Autodesk Fusion 360 part; units mm, degrees
note: some values were not read from the file. Set by a fixed rule: which sketch regions a step uses.
(part 6 of 15)
  line L4345 (-60.2725, -88.9984) -> (-60.4916, -88.82)
  line L4346 (182.212, -88.6982) -> (182.013, -88.8773)
  line L4347 (180.093, -85.6323) -> (180.347, -85.5433)
  line L4348 (-53.9287, -87.3136) -> (-53.7516, -87.3685)
  line L4349 (182.709, -87.7613) -> (182.636, -88.0196)
  line L4350 (182.744, -87.4953) -> (182.709, -87.7613)
  line L4351 (181.547, -89.1426) -> (181.292, -89.2235)
  line L4352 (181.891, -85.788) -> (182.104, -85.9508)
  line L4353 (181.789, -89.0264) -> (181.547, -89.1426)
  line L4354 (-58.9343, -89.3532) -> (-59.2167, -89.3599)
  line L4355 (181.657, -85.6568) -> (181.891, -85.788)
  line L4356 (182.636, -88.0196) -> (182.527, -88.2651)
  line L4357 (182.58, -86.5941) -> (182.673, -86.8459)
  line L4358 (-60.6018, -86.0161) -> (-60.3974, -85.8211)
  line L4359 (182.452, -86.3579) -> (182.58, -86.5941)
  line L4360 (182.293, -86.142) -> (182.452, -86.3579)
  line L4361 (-57.8967, -88.9424) -> (-58.1316, -89.0994)
  line L4362 (-58.1316, -89.0994) -> (-58.3863, -89.2216)
  line L4363 (182.527, -88.2651) -> (182.385, -88.4928)
  line L4364 (178.949, -87.3163) -> (178.976, -87.0493)
  line L4365 (-59.9168, -85.5266) -> (-59.6503, -85.433)
  line L4366 (-53.7516, -87.3685) -> (-53.5885, -87.4566)
  line L4367 (181.292, -89.2235) -> (181.027, -89.2676)
  line L4368 (-53.5885, -87.4566) -> (-53.4456, -87.5748)
  line L4369 (179.277, -86.308) -> (179.443, -86.0973)
  line L4370 (-61.0246, -86.7441) -> (-60.9186, -86.4822)
  line L4371 (182.673, -86.8459) -> (182.729, -87.1083)
  line L4372 (-58.3863, -89.2216) -> (-58.6556, -89.3068)
  line L4373 (-60.4916, -88.82) -> (-60.6834, -88.6126)
  line L4374 (182.385, -88.4928) -> (182.212, -88.6982)
  line L4375 (-59.2167, -89.3599) -> (-59.4973, -89.3267)
  line L4376 (182.013, -88.8773) -> (181.789, -89.0264)
  line L4377 (252.733, -84.9451) -> (252.831, -85.2102)
  line L4378 (252.792, -86.4456) -> (252.678, -86.704)
  line L4379 (-54.3237, -89.1721) -> (-54.5, -89.1148)
  line L4380 (-54.2977, -87.311) -> (-54.1131, -87.2942)
  line L4381 (251.901, -87.5054) -> (251.647, -87.6277)
  line L4382 (252.528, -86.9437) -> (252.347, -87.16)
  line L4383 (-53.6107, -89.0463) -> (-53.7762, -89.1299)
  line L4384 (-54.9182, -88.7588) -> (-55.003, -88.5939)
  line L4385 (249.541, -87.2261) -> (249.349, -87.0187)
  line L4386 (-54.7844, -87.5655) -> (-54.6399, -87.4493)
  line L4387 (249.349, -87.0187) -> (249.189, -86.7863)
  line L4388 (249.008, -85.1501) -> (249.114, -84.8883)
  line L4389 (252.136, -87.3485) -> (251.901, -87.5054)
  line L4390 (252.008, -84.0966) -> (252.233, -84.268)
  line L4391 (-54.5, -89.1148) -> (-54.6619, -89.0243)
  line L4392 (249.431, -84.4221) -> (249.635, -84.2271)
  line L4393 (249.865, -84.0629) -> (250.116, -83.9327)
  line L4394 (-55.0696, -88.231) -> (-55.0489, -88.0467)
  line L4395 (252.678, -86.704) -> (252.528, -86.9437)
  line L4396 (-53.3284, -87.7185) -> (-53.2414, -87.8822)
  line L4397 (252.831, -85.2102) -> (252.89, -85.4864)
  line L4398 (-54.4756, -87.3634) -> (-54.2977, -87.311)
  line L4399 (252.89, -85.4864) -> (252.91, -85.7682)
  line L4400 (-54.9929, -87.87) -> (-54.9036, -87.7075)
  line L4401 (251.498, -83.8566) -> (251.762, -83.9585)
  line L4402 (-54.6399, -87.4493) -> (-54.4756, -87.3634)
  line L4403 (251.377, -87.7129) -> (251.099, -87.7593)
  line L4404 (249.114, -84.8883) -> (249.256, -84.644)
  line L4405 (249.256, -84.644) -> (249.431, -84.4221)
  line L4406 (-53.2414, -87.8822) -> (-53.1878, -88.0597)
  line L4407 (248.922, -85.9876) -> (248.911, -85.7054)
  line L4408 (178.976, -87.0493) -> (179.041, -86.7889)
  line L4409 (252.869, -86.1737) -> (252.792, -86.4456)
  line L4410 (-53.1933, -88.4547) -> (-53.2518, -88.6306)
  line L4411 (-54.8031, -88.9041) -> (-54.9182, -88.7588)
  line L4412 (251.223, -83.7928) -> (251.498, -83.8566)
  line L4413 (251.647, -87.6277) -> (251.377, -87.7129)
  line L4414 (-53.1878, -88.0597) -> (-53.1697, -88.2442)
  line L4415 (-53.4456, -87.5748) -> (-53.3284, -87.7185)
  line L4416 (-55.0489, -88.0467) -> (-54.9929, -87.87)
  line L4417 (-55.0541, -88.4157) -> (-55.0696, -88.231)
  line L4418 (252.91, -85.7682) -> (252.906, -85.8938)
  line L4419 (252.906, -85.8938) -> (252.869, -86.1737)
  line L4420 (-54.6619, -89.0243) -> (-54.8031, -88.9041)
  line L4421 (251.762, -83.9585) -> (252.008, -84.0966)
  line L4422 (248.911, -85.7054) -> (248.94, -85.4243)
  line L4423 (-55.003, -88.5939) -> (-55.0541, -88.4157)
  line L4424 (-53.9547, -89.1798) -> (-54.1396, -89.194)
  line L4425 (252.431, -84.4693) -> (252.599, -84.6965)
  line L4426 (-54.9036, -87.7075) -> (-54.7844, -87.5655)
  line L4427 (248.94, -85.4243) -> (249.008, -85.1501)
  line L4428 (179.213, -88.3432) -> (179.093, -88.1031)
  line L4429 (-53.4646, -88.9322) -> (-53.6107, -89.0463)
  line L4430 (-53.7762, -89.1299) -> (-53.9547, -89.1798)
  line L4431 (-53.2518, -88.6306) -> (-53.3434, -88.7918)
  line L4432 (-53.1697, -88.2442) -> (-53.1701, -88.2707)
  line L4433 (180.347, -85.5433) -> (180.61, -85.491)
  line L4434 (252.233, -84.268) -> (252.431, -84.4693)
  line L4435 (252.599, -84.6965) -> (252.733, -84.9451)
  line L4436 (179.637, -85.912) -> (179.855, -85.756)
  line L4437 (-54.1131, -87.2942) -> (-53.9287, -87.3136)
  line L4438 (-53.1701, -88.2707) -> (-53.1933, -88.4547)
  line L4439 (-54.1396, -89.194) -> (-54.3237, -89.1721)
  line L4440 (85.4442, -85.7281) -> (85.4402, -85.8537)
  line L4441 (84.2957, -83.9185) -> (84.5422, -84.0565)
  line L4442 (82.5362, -87.5101) -> (82.2941, -87.3644)
  line L4443 (81.507, -86.2255) -> (81.4562, -85.9476)
  line L4444 (252.347, -87.16) -> (252.136, -87.3485)
  line L4445 (250.66, -83.7839) -> (250.942, -83.7684)
  line L4446 (84.8804, -87.1199) -> (84.67, -87.3084)
  line L4447 (249.063, -86.5335) -> (248.973, -86.2656)
  line L4448 (82.1693, -84.1871) -> (82.3992, -84.0228)
  line L4449 (251.099, -87.7593) -> (250.816, -87.766)
  line L4450 (81.5964, -86.4935) -> (81.507, -86.2255)
  line L4451 (246.072, -87.5859) -> (245.888, -87.6001)
  line L4452 (250.002, -87.5502) -> (249.76, -87.4045)
  line L4453 (246.684, -87.1979) -> (246.563, -87.3383)
  line L4454 (246.251, -87.536) -> (246.072, -87.5859)
  line L4455 (245.704, -87.5781) -> (245.527, -87.5209)
  line L4456 (245.365, -87.4304) -> (245.224, -87.3102)
  line L4457 (84.7668, -84.2279) -> (84.965, -84.4292)
  line L4458 (82.2941, -87.3644) -> (82.0751, -87.186)
  line L4459 (84.1804, -87.5877) -> (83.9111, -87.6728)
  line L4460 (85.267, -84.9051) -> (85.3647, -85.1701)
  line L4461 (85.4402, -85.8537) -> (85.4026, -86.1337)
  line L4462 (82.7963, -87.6203) -> (82.5362, -87.5101)
  line L4463 (84.4351, -87.4654) -> (84.1804, -87.5877)
  line L4464 (85.3647, -85.1701) -> (85.4242, -85.4463)
  line L4465 (249.189, -86.7863) -> (249.063, -86.5335)
  line L4466 (85.4026, -86.1337) -> (85.3259, -86.4056)
  line L4467 (85.0622, -86.9037) -> (84.8804, -87.1199)
  line L4468 (83.757, -83.7527) -> (84.0322, -83.8165)
  line L4469 (250.116, -83.9327) -> (250.383, -83.8391)
  line L4470 (84.5422, -84.0565) -> (84.7668, -84.2279)
  line L4471 (81.7227, -86.7462) -> (81.5964, -86.4935)
  line L4472 (84.965, -84.4292) -> (85.1328, -84.6565)
  line L4473 (246.834, -86.8608) -> (246.775, -87.0367)
  line L4474 (246.439, -85.8627) -> (246.582, -85.9809)
  line L4475 (83.9111, -87.6728) -> (83.6324, -87.7192)
  line L4476 (85.1328, -84.6565) -> (85.267, -84.9051)
  line L4477 (250.536, -87.7327) -> (250.263, -87.6603)
  line L4478 (250.263, -87.6603) -> (250.002, -87.5502)
  line L4479 (84.67, -87.3084) -> (84.4351, -87.4654)
  line L4480 (81.4451, -85.6653) -> (81.4739, -85.3842)
  line L4481 (85.2117, -86.664) -> (85.0622, -86.9037)
  line L4482 (81.6481, -84.8482) -> (81.79, -84.6039)
  line L4483 (246.699, -86.1246) -> (246.786, -86.2883)
  line L4484 (84.0322, -83.8165) -> (84.2957, -83.9185)
  line L4485 (250.942, -83.7684) -> (251.223, -83.7928)
  line L4486 (249.76, -87.4045) -> (249.541, -87.2261)
  line L4487 (85.4242, -85.4463) -> (85.4442, -85.7281)
  line L4488 (250.816, -87.766) -> (250.536, -87.7327)
  line L4489 (83.0694, -87.6927) -> (82.7963, -87.6203)
  line L4490 (83.3499, -87.7259) -> (83.0694, -87.6927)
  line L4491 (85.3259, -86.4056) -> (85.2117, -86.664)
  line L4492 (81.4562, -85.9476) -> (81.4451, -85.6653)
  line L4493 (83.6324, -87.7192) -> (83.3499, -87.7259)
  line L4494 (82.0751, -87.186) -> (81.8833, -86.9786)
  line L4495 (246.582, -85.9809) -> (246.699, -86.1246)
  line L4496 (81.9649, -84.3821) -> (82.1693, -84.1871)
  line L4497 (248.973, -86.2656) -> (248.922, -85.9876)
  line L4498 (81.8833, -86.9786) -> (81.7227, -86.7462)
  line L4499 (246.839, -86.4658) -> (246.858, -86.6503)
  line L4500 (249.635, -84.2271) -> (249.865, -84.0629)
  line L4501 (250.383, -83.8391) -> (250.66, -83.7839)
  line L4502 (89.3966, -86.6368) -> (89.3734, -86.8207)
  line L4503 (89.1211, -85.9408) -> (89.2383, -86.0845)
  line L4504 (245.527, -87.5209) -> (245.365, -87.4304)
  line L4505 (245.73, -85.7171) -> (245.914, -85.7003)
  line L4506 (81.542, -85.1101) -> (81.6481, -84.8482)
  line L4507 (244.973, -86.8218) -> (244.958, -86.637)
  line L4508 (89.1021, -87.2982) -> (88.956, -87.4124)
  line L4509 (245.109, -87.1649) -> (245.024, -87)
  line L4510 (245.224, -87.3102) -> (245.109, -87.1649)
  line L4511 (88.6119, -87.5458) -> (88.4271, -87.56)
  line L4512 (245.124, -86.1136) -> (245.243, -85.9716)
  line L4513 (83.1935, -83.7439) -> (83.4756, -83.7284)
  line L4514 (88.243, -87.5381) -> (88.0666, -87.4808)
  line L4515 (89.397, -86.6102) -> (89.3966, -86.6368)
  line L4516 (245.914, -85.7003) -> (246.099, -85.7197)
  line L4517 (244.958, -86.637) -> (244.978, -86.4528)
  line L4518 (88.8151, -85.7345) -> (88.9782, -85.8227)
  line L4519 (245.552, -85.7695) -> (245.73, -85.7171)
  line L4520 (89.2383, -86.0845) -> (89.3253, -86.2482)
  line L4521 (89.3789, -86.4257) -> (89.397, -86.6102)
  line L4522 (89.3148, -86.9966) -> (89.2233, -87.1579)
  line L4523 (82.6499, -83.8926) -> (82.9164, -83.799)
  line L4524 (87.9048, -87.3903) -> (87.7636, -87.2702)
  line L4525 (88.0666, -87.4808) -> (87.9048, -87.3903)
  line L4526 (-63.7818, -87.3657) -> (-63.9604, -87.4155)
  line L4527 (89.2233, -87.1579) -> (89.1021, -87.2982)
  line L4528 (88.956, -87.4124) -> (88.7905, -87.4959)
  line L4529 (88.7905, -87.4959) -> (88.6119, -87.5458)
  line L4530 (81.79, -84.6039) -> (81.9649, -84.3821)
  line L4531 (244.978, -86.4528) -> (245.034, -86.2761)
  line L4532 (-63.7572, -85.6042) -> (-63.5941, -85.6924)
  line L4533 (82.9164, -83.799) -> (83.1935, -83.7439)
  line L4534 (246.417, -87.4524) -> (246.251, -87.536)
  line L4535 (81.4739, -85.3842) -> (81.542, -85.1101)
  line L4536 (87.7636, -87.2702) -> (87.6484, -87.1249)
  line L4537 (-63.9604, -87.4155) -> (-64.1452, -87.4297)
  line L4538 (-64.1452, -87.4297) -> (-64.3293, -87.4078)
  line L4539 (245.387, -85.8554) -> (245.552, -85.7695)
  line L4540 (245.024, -87) -> (244.973, -86.8218)
  line L4541 (88.4271, -87.56) -> (88.243, -87.5381)
  line L4542 (-63.1757, -86.5065) -> (-63.199, -86.6904)
  line L4543 (87.6631, -86.0735) -> (87.7823, -85.9315)
  line L4544 (-63.199, -86.6904) -> (-63.2575, -86.8664)
  line L4545 (-63.6163, -87.2821) -> (-63.7818, -87.3657)
  line L4546 (88.638, -85.6796) -> (88.8151, -85.7345)
  line L4547 (246.857, -86.6768) -> (246.834, -86.8608)
  line L4548 (246.563, -87.3383) -> (246.417, -87.4524)
  line L4549 (246.099, -85.7197) -> (246.276, -85.7745)
  line L4550 (245.243, -85.9716) -> (245.387, -85.8554)
  line L4551 (88.9782, -85.8227) -> (89.1211, -85.9408)
  line L4552 (-64.3293, -87.4078) -> (-64.5057, -87.3505)
  line L4553 (-64.5057, -87.3505) -> (-64.6675, -87.26)
  line L4554 (245.888, -87.6001) -> (245.704, -87.5781)
  line L4555 (89.3734, -86.8207) -> (89.3148, -86.9966)
  line L4556 (-63.9343, -85.5494) -> (-63.7572, -85.6042)
  line L4557 (87.5126, -86.7817) -> (87.4971, -86.597)
  line L4558 (246.775, -87.0367) -> (246.684, -87.1979)
  line L4559 (82.3992, -84.0228) -> (82.6499, -83.8926)
  line L4560 (245.034, -86.2761) -> (245.124, -86.1136)
  line L4561 (246.858, -86.6503) -> (246.857, -86.6768)
  line L4562 (246.276, -85.7745) -> (246.439, -85.8627)
  line L4563 (83.4756, -83.7284) -> (83.757, -83.7527)
  line L4564 (89.3253, -86.2482) -> (89.3789, -86.4257)
  line L4565 (246.786, -86.2883) -> (246.839, -86.4658)
  line L4566 (270.656, -82.7999) -> (270.919, -82.9018)
  line L4567 (-64.1187, -85.53) -> (-63.9343, -85.5494)
  line L4568 (271.391, -83.2112) -> (271.589, -83.4125)
  line L4569 (268.131, -85.2088) -> (268.08, -84.9309)
  line L4570 (272.064, -84.837) -> (272.026, -85.117)
  line L4571 (271.686, -85.887) -> (271.504, -86.1033)
  line L4572 (-63.3341, -85.9542) -> (-63.247, -86.1179)
  line L4573 (65.1382, -82.8617) -> (65.3847, -82.9998)
  line L4574 (-64.9985, -86.1057) -> (-64.9092, -85.9432)
  line L4575 (-65.0086, -86.8297) -> (-65.0597, -86.6514)
  line L4576 (268.08, -84.9309) -> (268.069, -84.6486)
  line L4577 (-64.3034, -85.5468) -> (-64.1187, -85.53)
  line L4578 (270.099, -82.7117) -> (270.381, -82.7361)
  line L4579 (65.3847, -82.9998) -> (65.6092, -83.1712)
  line L4580 (87.9268, -85.8153) -> (88.0911, -85.7294)
  line L4581 (272.026, -85.117) -> (271.95, -85.3889)
  line L4582 (-65.0753, -86.4667) -> (-65.0546, -86.2824)
  line L4583 (-63.2575, -86.8664) -> (-63.3491, -87.0276)
  line L4584 (87.7823, -85.9315) -> (87.9268, -85.8153)
  line L4585 (88.4536, -85.6603) -> (88.638, -85.6796)
  line L4586 (271.891, -83.8884) -> (271.988, -84.1535)
  line L4587 (-64.9092, -85.9432) -> (-64.79, -85.8012)
  line L4588 (64.5995, -82.696) -> (64.8747, -82.7598)
  line L4589 (269.693, -86.676) -> (269.42, -86.6036)
  line L4590 (-63.5941, -85.6924) -> (-63.4513, -85.8106)
  line L4591 (268.918, -86.3477) -> (268.699, -86.1694)
  line L4592 (271.504, -86.1033) -> (271.294, -86.2918)
  line L4593 (270.256, -86.7026) -> (269.974, -86.7092)
  line L4594 (-64.79, -85.8012) -> (-64.6455, -85.685)
  line L4595 (-64.6675, -87.26) -> (-64.8087, -87.1399)
  line L4596 (-63.4513, -85.8106) -> (-63.3341, -85.9542)
  line L4597 (87.4971, -86.597) -> (87.5177, -86.4127)
  line L4598 (87.5738, -86.236) -> (87.6631, -86.0735)
  line L4599 (87.6484, -87.1249) -> (87.5637, -86.96)
  line L4600 (-64.8087, -87.1399) -> (-64.9239, -86.9946)
  line L4601 (-64.9239, -86.9946) -> (-65.0086, -86.8297)
  line L4602 (87.5177, -86.4127) -> (87.5738, -86.236)
  line L4603 (-65.0546, -86.2824) -> (-64.9985, -86.1057)
  line L4604 (272.048, -84.4296) -> (272.068, -84.7114)
  line L4605 (271.294, -86.2918) -> (271.059, -86.4487)
  line L4606 (269.42, -86.6036) -> (269.16, -86.4935)
  line L4607 (271.95, -85.3889) -> (271.835, -85.6473)
  line L4608 (-63.1753, -86.48) -> (-63.1757, -86.5065)
  line L4609 (88.269, -85.6771) -> (88.4536, -85.6603)
  line L4610 (88.0911, -85.7294) -> (88.269, -85.6771)
  line L4611 (-63.4702, -87.1679) -> (-63.6163, -87.2821)
  line L4612 (271.757, -83.6398) -> (271.891, -83.8884)
  line L4613 (270.381, -82.7361) -> (270.656, -82.7999)
  line L4614 (-63.247, -86.1179) -> (-63.1934, -86.2954)
  line L4615 (270.919, -82.9018) -> (271.166, -83.0398)
  line L4616 (272.068, -84.7114) -> (272.064, -84.837)
  line L4617 (271.835, -85.6473) -> (271.686, -85.887)
  line L4618 (-65.0597, -86.6514) -> (-65.0753, -86.4667)
  line L4619 (271.988, -84.1535) -> (272.048, -84.4296)
  line L4620 (-63.1934, -86.2954) -> (-63.1753, -86.48)
  line L4621 (268.272, -83.8316) -> (268.414, -83.5873)
  line L4622 (64.8747, -82.7598) -> (65.1382, -82.8617)
  line L4623 (271.166, -83.0398) -> (271.391, -83.2112)
  line L4624 (269.274, -82.8759) -> (269.54, -82.7823)
  line L4625 (271.589, -83.4125) -> (271.757, -83.6398)
  line L4626 (-63.3491, -87.0276) -> (-63.4702, -87.1679)
  line L4627 (87.5637, -86.96) -> (87.5126, -86.7817)
  line L4628 (-64.4812, -85.5991) -> (-64.3034, -85.5468)
  line L4629 (-64.6455, -85.685) -> (-64.4812, -85.5991)
  line L4630 (66.2072, -84.1134) -> (66.2667, -84.3896)
  line L4631 (269.817, -82.7272) -> (270.099, -82.7117)
  line L4632 (63.1366, -86.3077) -> (62.9175, -86.1293)
  line L4633 (62.4389, -85.4367) -> (62.3494, -85.1688)
  line L4634 (62.5651, -85.6895) -> (62.4389, -85.4367)
  line L4635 (268.346, -85.7295) -> (268.22, -85.4768)
  line L4636 (270.804, -86.571) -> (270.535, -86.6562)
  line L4637 (65.6092, -83.1712) -> (65.8074, -83.3725)
  line L4638 (270.535, -86.6562) -> (270.256, -86.7026)
  line L4639 (65.9753, -83.5997) -> (66.1094, -83.8484)
  line L4640 (62.4906, -83.7915) -> (62.6324, -83.5472)
  line L4641 (65.8074, -83.3725) -> (65.9753, -83.5997)
  line L4642 (66.1094, -83.8484) -> (66.2072, -84.1134)
  line L4643 (268.22, -85.4768) -> (268.131, -85.2088)
  line L4644 (62.3164, -84.3275) -> (62.3845, -84.0533)
  line L4645 (66.2451, -85.077) -> (66.1684, -85.3489)
  line L4646 (66.0541, -85.6072) -> (65.9046, -85.847)
  line L4647 (64.1924, -86.6692) -> (63.9118, -86.636)
  line L4648 (62.3845, -84.0533) -> (62.4906, -83.7915)
  line L4649 (62.3494, -85.1688) -> (62.2987, -84.8908)
  line L4650 (64.7535, -86.6161) -> (64.4748, -86.6625)
  line L4651 (271.059, -86.4487) -> (270.804, -86.571)
  line L4652 (62.6324, -83.5472) -> (62.8073, -83.3254)
  line L4653 (265.256, -84.663) -> (265.433, -84.7178)
  line L4654 (65.9046, -85.847) -> (65.7229, -86.0632)
  line L4655 (64.4748, -86.6625) -> (64.1924, -86.6692)
  line L4656 (268.069, -84.6486) -> (268.098, -84.3676)
  line L4657 (268.793, -83.1704) -> (269.023, -83.0062)
  line L4658 (62.8073, -83.3254) -> (63.0118, -83.1304)
  line L4659 (63.4923, -82.8359) -> (63.7589, -82.7423)
  line L4660 (62.2987, -84.8908) -> (62.2876, -84.6086)
  line L4661 (65.7229, -86.0632) -> (65.5124, -86.2517)
  line L4662 (66.2866, -84.6714) -> (66.2827, -84.797)
  line L4663 (63.3786, -86.4534) -> (63.1366, -86.3077)
  line L4664 (265.841, -86.1412) -> (265.72, -86.2815)
  line L4665 (265.72, -86.2815) -> (265.574, -86.3957)
  line L4666 (62.7257, -85.9219) -> (62.5651, -85.6895)
  line L4667 (268.414, -83.5873) -> (268.589, -83.3654)
  line L4668 (269.974, -86.7092) -> (269.693, -86.676)
  line L4669 (65.0229, -86.5309) -> (64.7535, -86.6161)
  line L4670 (65.2775, -86.4086) -> (65.0229, -86.5309)
  line L4671 (66.2667, -84.3896) -> (66.2866, -84.6714)
  line L4672 (66.1684, -85.3489) -> (66.0541, -85.6072)
  line L4673 (63.9118, -86.636) -> (63.6388, -86.5636)
  line L4674 (66.2827, -84.797) -> (66.2451, -85.077)
  line L4675 (268.098, -84.3676) -> (268.166, -84.0934)
  line L4676 (268.507, -85.9619) -> (268.346, -85.7295)
  line L4677 (62.2876, -84.6086) -> (62.3164, -84.3275)
  line L4678 (62.9175, -86.1293) -> (62.7257, -85.9219)
  line L4679 (265.409, -86.4793) -> (265.23, -86.5291)
  line L4680 (64.318, -82.6716) -> (64.5995, -82.696)
  line L4681 (265.997, -85.4091) -> (266.015, -85.5936)
  line L4682 (64.0359, -82.6872) -> (64.318, -82.6716)
  line L4683 (269.16, -86.4935) -> (268.918, -86.3477)
  line L4684 (63.2416, -82.9661) -> (63.4923, -82.8359)
  line L4685 (264.685, -86.4641) -> (264.523, -86.3737)
  line L4686 (269.54, -82.7823) -> (269.817, -82.7272)
  line L4687 (264.523, -86.3737) -> (264.382, -86.2535)
  line L4688 (65.5124, -86.2517) -> (65.2775, -86.4086)
  line L4689 (63.6388, -86.5636) -> (63.3786, -86.4534)
  line L4690 (268.699, -86.1694) -> (268.507, -85.9619)
  line L4691 (268.166, -84.0934) -> (268.272, -83.8316)
  line L4692 (268.589, -83.3654) -> (268.793, -83.1704)
  line L4693 (269.023, -83.0062) -> (269.274, -82.8759)
  line L4694 (265.856, -85.0679) -> (265.943, -85.2316)
  line L4695 (265.991, -85.804) -> (265.933, -85.98)
  line L4696 (265.23, -86.5291) -> (265.045, -86.5434)
  line L4697 (265.933, -85.98) -> (265.841, -86.1412)
  line L4698 (63.0118, -83.1304) -> (63.2416, -82.9661)
  line L4699 (265.943, -85.2316) -> (265.997, -85.4091)
  line L4700 (266.015, -85.5936) -> (266.015, -85.6201)
  line L4701 (68.4061, -85.9032) -> (68.355, -85.725)
  line L4702 (69.8207, -84.7659) -> (69.9635, -84.8841)
  line L4703 (70.2213, -85.369) -> (70.2394, -85.5535)
  line L4704 (264.136, -85.3961) -> (264.192, -85.2193)
  line L4705 (70.1678, -85.1915) -> (70.2213, -85.369)
  line L4706 (264.115, -85.5803) -> (264.136, -85.3961)
  line L4707 (265.072, -84.6436) -> (265.256, -84.663)
  line L4708 (68.6061, -86.2134) -> (68.4909, -86.0681)
  line L4709 (69.633, -86.4392) -> (69.4544, -86.4891)
  line L4710 (69.2695, -86.5033) -> (69.0854, -86.4814)
  line L4711 (70.0657, -86.1011) -> (69.9446, -86.2415)
  line L4712 (70.2394, -85.5535) -> (70.2391, -85.58)
  line L4713 (264.4, -84.9148) -> (264.545, -84.7987)
  line L4714 (264.709, -84.7128) -> (264.887, -84.6604)
  line L4715 (68.6248, -84.8748) -> (68.7692, -84.7586)
  line L4716 (289.902, -82.2434) -> (290.165, -82.3453)
  line L4717 (290.636, -82.6548) -> (290.834, -82.8561)
  line L4718 (69.6576, -84.6777) -> (69.8207, -84.7659)
  line L4719 (265.045, -86.5434) -> (264.861, -86.5214)
  line L4720 (68.355, -85.725) -> (68.3395, -85.5402)
  line L4721 (290.932, -85.3306) -> (290.75, -85.5468)
  line L4722 (70.2158, -85.764) -> (70.1573, -85.9399)
  line L4723 (291.002, -83.0833) -> (291.136, -83.332)
  line L4724 (264.281, -85.0569) -> (264.4, -84.9148)
  line L4725 (69.9446, -86.2415) -> (69.7985, -86.3556)
  line L4726 (68.9091, -86.4241) -> (68.7473, -86.3336)
  line L4727 (70.0807, -85.0278) -> (70.1678, -85.1915)
  line L4728 (264.545, -84.7987) -> (264.709, -84.7128)
  line L4729 (70.2391, -85.58) -> (70.2158, -85.764)
  line L4730 (69.0854, -86.4814) -> (68.9091, -86.4241)
  line L4731 (68.4163, -85.1793) -> (68.5056, -85.0168)
  line L4732 (290.834, -82.8561) -> (291.002, -83.0833)
  line L4733 (63.7589, -82.7423) -> (64.0359, -82.6872)
  line L4734 (265.433, -84.7178) -> (265.596, -84.806)
  line L4735 (266.015, -85.6201) -> (265.991, -85.804)
  line L4736 (69.4544, -86.4891) -> (69.2695, -86.5033)
  line L4737 (69.9635, -84.8841) -> (70.0807, -85.0278)
  line L4738 (264.887, -84.6604) -> (265.072, -84.6436)
  line L4739 (265.739, -84.9242) -> (265.856, -85.0679)
  line L4740 (69.4805, -84.6229) -> (69.6576, -84.6777)
  line L4741 (70.1573, -85.9399) -> (70.0657, -86.1011)
  line L4742 (264.192, -85.2193) -> (264.281, -85.0569)
  line L4743 (289.502, -86.1461) -> (289.219, -86.1528)
  line L4744 (68.3602, -85.356) -> (68.4163, -85.1793)
  line L4745 (69.1114, -84.6203) -> (69.2961, -84.6035)
  line L4746 (69.7985, -86.3556) -> (69.633, -86.4392)
  line L4747 (265.574, -86.3957) -> (265.409, -86.4793)
  line L4748 (68.4909, -86.0681) -> (68.4061, -85.9032)
  line L4749 (289.627, -82.1796) -> (289.902, -82.2434)
  line L4750 (290.165, -82.3453) -> (290.412, -82.4834)
  line L4751 (68.7473, -86.3336) -> (68.6061, -86.2134)
  line L4752 (264.861, -86.5214) -> (264.685, -86.4641)
  line L4753 (264.131, -85.7651) -> (264.115, -85.5803)
  line L4754 (264.382, -86.2535) -> (264.267, -86.1082)
  line L4755 (264.267, -86.1082) -> (264.182, -85.9433)
  line L4756 (264.182, -85.9433) -> (264.131, -85.7651)
  line L4757 (265.596, -84.806) -> (265.739, -84.9242)
  line L4758 (45.8924, -82.3053) -> (46.1389, -82.4433)
  line L4759 (287.343, -83.8111) -> (287.412, -83.537)
  line L4760 (46.1389, -82.4433) -> (46.3635, -82.6147)
  line L4761 (45.5077, -86.0597) -> (45.2291, -86.1061)
  line L4762 (291.234, -83.597) -> (291.294, -83.8732)
  line L4763 (287.412, -83.537) -> (287.518, -83.2751)
  line L4764 (46.5617, -82.816) -> (46.7295, -83.0433)
  line L4765 (290.539, -85.7353) -> (290.305, -85.8923)
  line L4766 (46.8637, -83.2919) -> (46.9614, -83.557)
  line L4767 (68.5056, -85.0168) -> (68.6248, -84.8748)
  line L4768 (47.0209, -83.8331) -> (47.0409, -84.1149)
  line L4769 (46.9226, -84.7924) -> (46.8084, -85.0508)
  line L4770 (43.0706, -83.7711) -> (43.1387, -83.4969)
  line L4771 (288.519, -82.3195) -> (288.786, -82.2259)
  line L4772 (43.2448, -83.2351) -> (43.3867, -82.9908)
  line L4773 (287.945, -85.6129) -> (287.753, -85.4055)
  line L4774 (288.269, -82.4497) -> (288.519, -82.3195)
  line L4775 (43.3194, -85.133) -> (43.1931, -84.8803)
  line L4776 (291.195, -84.8325) -> (291.081, -85.0909)
  line L4777 (43.1037, -84.6123) -> (43.0529, -84.3344)
  line L4778 (46.7295, -83.0433) -> (46.8637, -83.2919)
  line L4779 (287.834, -82.809) -> (288.039, -82.614)
  line L4780 (290.05, -86.0146) -> (289.781, -86.0997)
  line L4781 (289.219, -86.1528) -> (288.939, -86.1196)
  line L4782 (289.063, -82.1708) -> (289.345, -82.1552)
  line L4783 (287.518, -83.2751) -> (287.659, -83.0308)
  line L4784 (45.3537, -82.1396) -> (45.6289, -82.2033)
  line L4785 (43.48, -85.3654) -> (43.3194, -85.133)
  line L4786 (68.9336, -84.6727) -> (69.1114, -84.6203)
  line L4787 (287.315, -84.0922) -> (287.343, -83.8111)
  line L4788 (288.939, -86.1196) -> (288.666, -86.0472)
  line L4789 (291.136, -83.332) -> (291.234, -83.597)
  line L4790 (291.314, -84.155) -> (291.31, -84.2806)
  line L4791 (287.659, -83.0308) -> (287.834, -82.809)
  line L4792 (68.7692, -84.7586) -> (68.9336, -84.6727)
  line L4793 (288.786, -82.2259) -> (289.063, -82.1708)
  line L4794 (44.1329, -85.8969) -> (43.8908, -85.7512)
  line L4795 (288.406, -85.937) -> (288.164, -85.7913)
  line L4796 (290.75, -85.5468) -> (290.539, -85.7353)
  line L4797 (291.081, -85.0909) -> (290.932, -85.3306)
  line L4798 (287.376, -84.6524) -> (287.326, -84.3745)
  line L4799 (45.6289, -82.2033) -> (45.8924, -82.3053)
  line L4800 (46.3635, -82.6147) -> (46.5617, -82.816)
  line L4801 (290.305, -85.8923) -> (290.05, -86.0146)
  line L4802 (287.466, -84.9204) -> (287.376, -84.6524)
  line L4803 (68.3395, -85.5402) -> (68.3602, -85.356)
  line L4804 (290.412, -82.4834) -> (290.636, -82.6548)
  line L4805 (287.326, -84.3745) -> (287.315, -84.0922)
  line L4806 (287.592, -85.1731) -> (287.466, -84.9204)
  line L4807 (291.294, -83.8732) -> (291.314, -84.155)
  line L4808 (288.164, -85.7913) -> (287.945, -85.6129)
  line L4809 (288.039, -82.614) -> (288.269, -82.4497)
  line L4810 (287.753, -85.4055) -> (287.592, -85.1731)
  line L4811 (43.6718, -85.5729) -> (43.48, -85.3654)
  line L4812 (46.4771, -85.5068) -> (46.2667, -85.6952)
  line L4813 (44.393, -86.0071) -> (44.1329, -85.8969)
  line L4814 (289.345, -82.1552) -> (289.627, -82.1796)
  line L4815 (43.0529, -84.3344) -> (43.0418, -84.0521)
  line L4816 (291.31, -84.2806) -> (291.272, -84.5606)
  line L4817 (288.666, -86.0472) -> (288.406, -85.937)
  line L4818 (46.9614, -83.557) -> (47.0209, -83.8331)
  line L4819 (291.272, -84.5606) -> (291.195, -84.8325)
  line L4820 (69.2961, -84.6035) -> (69.4805, -84.6229)
  line L4821 (289.781, -86.0997) -> (289.502, -86.1461)
  line L4822 (47.0369, -84.2405) -> (46.9993, -84.5205)
  line L4823 (284.502, -84.1065) -> (284.679, -84.1614)
  line L4824 (285.261, -85.0371) -> (285.26, -85.0637)
  line L4825 (285.243, -84.8526) -> (285.261, -85.0371)
  line L4826 (43.9959, -82.4097) -> (44.2466, -82.2794)
  line L4827 (43.1931, -84.8803) -> (43.1037, -84.6123)
  line L4828 (45.2291, -86.1061) -> (44.9466, -86.1127)
  line L4829 (46.6589, -85.2905) -> (46.4771, -85.5068)
  line L4830 (46.8084, -85.0508) -> (46.6589, -85.2905)
  line L4831 (285.189, -84.6751) -> (285.243, -84.8526)
  line L4832 (44.7902, -82.1307) -> (45.0723, -82.1152)
  line L4833 (283.512, -85.5518) -> (283.428, -85.3869)
  line L4834 (283.428, -85.3869) -> (283.376, -85.2086)
  line L4835 (283.527, -84.5004) -> (283.646, -84.3584)
  line L4836 (285.087, -85.5847) -> (284.966, -85.7251)
  line L4837 (284.291, -85.9869) -> (284.107, -85.965)
  line L4838 (283.769, -85.8172) -> (283.627, -85.6971)
  line L4839 (46.0318, -85.8522) -> (45.7771, -85.9745)
  line L4840 (283.627, -85.6971) -> (283.512, -85.5518)
  line L4841 (44.2466, -82.2794) -> (44.5131, -82.1858)
  line L4842 (45.0723, -82.1152) -> (45.3537, -82.1396)
  line L4843 (44.9466, -86.1127) -> (44.6661, -86.0795)
  line L4844 (43.1387, -83.4969) -> (43.2448, -83.2351)
  line L4845 (284.82, -85.8392) -> (284.654, -85.9228)
  line L4846 (284.654, -85.9228) -> (284.476, -85.9727)
  line L4847 (284.966, -85.7251) -> (284.82, -85.8392)
  line L4848 (284.107, -85.965) -> (283.93, -85.9077)
  line L4849 (284.842, -84.2495) -> (284.985, -84.3677)
  line L4850 (284.679, -84.1614) -> (284.842, -84.2495)
  line L4851 (283.376, -85.2086) -> (283.361, -85.0239)
  line L4852 (43.5616, -82.7689) -> (43.766, -82.5739)
  line L4853 (47.0409, -84.1149) -> (47.0369, -84.2405)
  line L4854 (285.26, -85.0637) -> (285.237, -85.2476)
  line L4855 (44.5131, -82.1858) -> (44.7902, -82.1307)
  line L4856 (284.985, -84.3677) -> (285.102, -84.5114)
  line L4857 (285.237, -85.2476) -> (285.179, -85.4235)
  line L4858 (283.93, -85.9077) -> (283.769, -85.8172)
  line L4859 (43.3867, -82.9908) -> (43.5616, -82.7689)
  line L4860 (43.0418, -84.0521) -> (43.0706, -83.7711)
  line L4861 (285.179, -85.4235) -> (285.087, -85.5847)
  line L4862 (285.102, -84.5114) -> (285.189, -84.6751)
  line L4863 (284.476, -85.9727) -> (284.291, -85.9869)
  line L4864 (283.438, -84.6629) -> (283.527, -84.5004)
  line L4865 (43.766, -82.5739) -> (43.9959, -82.4097)
  line L4866 (283.361, -85.0239) -> (283.382, -84.8396)
  line L4867 (50.922, -84.6351) -> (50.9756, -84.8125)
  line L4868 (50.9756, -84.8125) -> (50.9937, -84.9971)
  line L4869 (283.382, -84.8396) -> (283.438, -84.6629)
  line L4870 (43.8908, -85.7512) -> (43.6718, -85.5729)
  line L4871 (44.6661, -86.0795) -> (44.393, -86.0071)
  line L4872 (46.2667, -85.6952) -> (46.0318, -85.8522)
  line L4873 (45.7771, -85.9745) -> (45.5077, -86.0597)
  line L4874 (46.9993, -84.5205) -> (46.9226, -84.7924)
  line L4875 (-4.7396, -78.5712) -> (-4.9159, -78.5139)
  line L4876 (-4.3446, -76.7128) -> (-4.1674, -76.7676)
  line L4877 (-3.5859, -77.6699) -> (-3.6092, -77.8538)
  line L4878 (216.669, -76.7183) -> (216.756, -76.882)
  line L4879 (216.387, -78.0461) -> (216.221, -78.1297)
  line L4880 (215.195, -77.9039) -> (215.079, -77.7586)
  line L4881 (214.949, -77.0465) -> (215.005, -76.8697)
  line L4882 (216.828, -77.2705) -> (216.804, -77.4545)
  line L4883 (216.552, -76.5746) -> (216.669, -76.7183)
  line L4884 (214.995, -77.5937) -> (214.944, -77.4155)
  line L4885 (216.756, -76.882) -> (216.81, -77.0595)
  line L4886 (216.828, -77.244) -> (216.828, -77.2705)
  line L4887 (-5.2003, -76.9646) -> (-5.0558, -76.8484)
  line L4888 (216.069, -76.3134) -> (216.246, -76.3682)
  line L4889 (215.336, -78.0241) -> (215.195, -77.9039)
  line L4890 (216.81, -77.0595) -> (216.828, -77.244)
  line L4891 (215.858, -78.1938) -> (215.674, -78.1718)
  line L4892 (-3.8804, -78.3313) -> (-4.0266, -78.4455)
  line L4893 (216.654, -77.7916) -> (216.533, -77.932)
  line L4894 (-3.6677, -78.0298) -> (-3.7593, -78.191)
  line L4895 (215.079, -77.7586) -> (214.995, -77.5937)
  line L4896 (215.674, -78.1718) -> (215.498, -78.1145)
  line L4897 (216.533, -77.932) -> (216.387, -78.0461)
  line L4898 (-5.4088, -77.2691) -> (-5.3194, -77.1066)
  line L4899 (-5.3194, -77.1066) -> (-5.2003, -76.9646)
  line L4900 (-5.4648, -77.4458) -> (-5.4088, -77.2691)
  line L4901 (-3.8615, -76.974) -> (-3.7443, -77.1176)
  line L4902 (216.221, -78.1297) -> (216.043, -78.1796)
  line L4903 (-4.7136, -76.7102) -> (-4.529, -76.6934)
  line L4904 (216.043, -78.1796) -> (215.858, -78.1938)
  line L4905 (215.498, -78.1145) -> (215.336, -78.0241)
  line L4906 (216.804, -77.4545) -> (216.746, -77.6304)
  line L4907 (216.409, -76.4564) -> (216.552, -76.5746)
  line L4908 (117.527, -77.1907) -> (117.547, -77.0064)
  line L4909 (-5.0558, -76.8484) -> (-4.8915, -76.7625)
  line L4910 (118.845, -76.3282) -> (119.008, -76.4163)
  line L4911 (119.151, -76.5345) -> (119.268, -76.6782)
  line L4912 (216.246, -76.3682) -> (216.409, -76.4564)
  line L4913 (128.489, -78.0182) -> (128.673, -78.0376)
  line L4914 (216.746, -77.6304) -> (216.654, -77.7916)
  line L4915 (214.928, -77.2307) -> (214.949, -77.0465)
  line L4916 (-5.47, -77.8149) -> (-5.4855, -77.6301)
  line L4917 (119.253, -77.7515) -> (119.132, -77.8919)
  line L4918 (-4.529, -76.6934) -> (-4.3446, -76.7128)
  line L4919 (-4.0266, -78.4455) -> (-4.192, -78.5291)
  line L4920 (-4.8915, -76.7625) -> (-4.7136, -76.7102)
  line L4921 (118.82, -78.0896) -> (118.642, -78.1395)
  line L4922 (214.944, -77.4155) -> (214.928, -77.2307)
  line L4923 (-5.4189, -77.9931) -> (-5.47, -77.8149)
  line L4924 (-4.5555, -78.5932) -> (-4.7396, -78.5712)
  line L4925 (-4.9159, -78.5139) -> (-5.0778, -78.4235)
  line L4926 (-4.192, -78.5291) -> (-4.3706, -78.5789)
  line L4927 (-3.6037, -77.4588) -> (-3.5856, -77.6434)
  line L4928 (-4.3706, -78.5789) -> (-4.5555, -78.5932)
  line L4929 (-4.0043, -76.8558) -> (-3.8615, -76.974)
  line L4930 (128.126, -78.0874) -> (128.304, -78.035)
  line L4931 (127.818, -78.2894) -> (127.962, -78.1733)
  line L4932 (-3.6573, -77.2813) -> (-3.6037, -77.4588)
  line L4933 (-3.7443, -77.1176) -> (-3.6573, -77.2813)
  line L4934 (127.962, -78.1733) -> (128.126, -78.0874)
  line L4935 (-5.3341, -78.158) -> (-5.4189, -77.9931)
  line L4936 (-3.7593, -78.191) -> (-3.8804, -78.3313)
  line L4937 (-5.4855, -77.6301) -> (-5.4648, -77.4458)
  line L4938 (-5.0778, -78.4235) -> (-5.219, -78.3033)
  line L4939 (118.668, -76.2733) -> (118.845, -76.3282)
  line L4940 (119.132, -77.8919) -> (118.986, -78.006)
  line L4941 (118.642, -78.1395) -> (118.457, -78.1537)
  line L4942 (118.096, -78.0745) -> (117.934, -77.984)
  line L4943 (-16.5258, -76.1534) -> (-16.6753, -76.3931)
  line L4944 (-17.9805, -73.2421) -> (-17.7053, -73.3059)
  line L4945 (118.121, -76.3231) -> (118.299, -76.2707)
  line L4946 (-17.4418, -73.4078) -> (-17.1953, -73.5459)
  line L4947 (-16.3349, -75.6231) -> (-16.4116, -75.895)
  line L4948 (-16.3133, -74.9357) -> (-16.2933, -75.2175)
  line L4949 (118.457, -78.1537) -> (118.273, -78.1318)
  line L4950 (118.483, -76.2539) -> (118.668, -76.2733)
  line L4951 (-17.3024, -76.9548) -> (-17.5571, -77.0771)
  line L4952 (215.885, -76.294) -> (216.069, -76.3134)
  line L4953 (-17.1953, -73.5459) -> (-16.9707, -73.7173)
  line L4954 (215.522, -76.3632) -> (215.7, -76.3108)
  line L4955 (118.273, -78.1318) -> (118.096, -78.0745)
  line L4956 (119.008, -76.4163) -> (119.151, -76.5345)
  line L4957 (-18.3876, -77.2153) -> (-18.6681, -77.1821)
  line L4958 (-16.6753, -76.3931) -> (-16.8571, -76.6093)
  line L4959 (-17.5571, -77.0771) -> (-17.8265, -77.1622)
  line L4960 (117.934, -77.984) -> (117.793, -77.8638)
  line L4961 (117.812, -76.5252) -> (117.956, -76.409)
  line L4962 (117.603, -76.8297) -> (117.693, -76.6672)
  line L4963 (-16.3728, -74.6595) -> (-16.3133, -74.9357)
  line L4964 (-18.1051, -77.2086) -> (-18.3876, -77.2153)
  line L4965 (119.355, -76.8419) -> (119.408, -77.0194)
  line L4966 (-16.8571, -76.6093) -> (-17.0675, -76.7978)
  line L4967 (215.213, -76.5652) -> (215.358, -76.4491)
  line L4968 (119.408, -77.0194) -> (119.427, -77.2039)
  line L4969 (119.403, -77.4144) -> (119.344, -77.5903)
  line L4970 (117.793, -77.8638) -> (117.678, -77.7185)
  line L4971 (117.547, -77.0064) -> (117.603, -76.8297)
  line L4972 (-16.4705, -74.3945) -> (-16.3728, -74.6595)
  line L4973 (-18.9412, -77.1097) -> (-19.2013, -76.9995)
  line L4974 (-20.2305, -75.7149) -> (-20.2813, -75.437)
  line L4975 (-20.1411, -75.9829) -> (-20.2305, -75.7149)
  line L4976 (-16.2973, -75.3431) -> (-16.3349, -75.6231)
  line L4977 (-16.7725, -73.9186) -> (-16.6047, -74.1458)
  line L4978 (117.542, -77.3754) -> (117.527, -77.1907)
  line L4979 (-18.6681, -77.1821) -> (-18.9412, -77.1097)
  line L4980 (-16.6047, -74.1458) -> (-16.4705, -74.3945)
  line L4981 (-19.7726, -73.8715) -> (-19.5682, -73.6765)
  line L4982 (-18.544, -73.2333) -> (-18.2619, -73.2177)
  line L4983 (118.986, -78.006) -> (118.82, -78.0896)
  line L4984 (-16.4116, -75.895) -> (-16.5258, -76.1534)
  line L4985 (119.427, -77.2039) -> (119.426, -77.2304)
  line L4986 (215.7, -76.3108) -> (215.885, -76.294)
  line L4987 (117.693, -76.6672) -> (117.812, -76.5252)
  line L4988 (-16.9707, -73.7173) -> (-16.7725, -73.9186)
  line L4989 (-16.2933, -75.2175) -> (-16.2973, -75.3431)
  line L4990 (-17.0675, -76.7978) -> (-17.3024, -76.9548)
  line L4991 (-17.8265, -77.1622) -> (-18.1051, -77.2086)
  line L4992 (117.956, -76.409) -> (118.121, -76.3231)
  line L4993 (118.299, -76.2707) -> (118.483, -76.2539)
  line L4994 (-17.7053, -73.3059) -> (-17.4418, -73.4078)
  line L4995 (117.678, -77.7185) -> (117.593, -77.5536)
  line L4996 (119.344, -77.5903) -> (119.253, -77.7515)
  line L4997 (119.426, -77.2304) -> (119.403, -77.4144)
  line L4998 (215.005, -76.8697) -> (215.094, -76.7073)
  line L4999 (215.358, -76.4491) -> (215.522, -76.3632)
  line L5000 (215.094, -76.7073) -> (215.213, -76.5652)
  line L5001 (117.593, -77.5536) -> (117.542, -77.3754)
  line L5002 (119.268, -76.6782) -> (119.355, -76.8419)
  line L5003 (-20.2924, -75.1547) -> (-20.2636, -74.8736)
  line L5004 (-12.3405, -76.0996) -> (-12.3409, -76.1262)
  line L5005 (-12.6164, -75.4302) -> (-12.4992, -75.5739)
  line L5006 (-19.5682, -73.6765) -> (-19.3383, -73.5122)
  line L5007 (-12.3586, -75.9151) -> (-12.3405, -76.0996)
  line L5008 (-12.3641, -76.3101) -> (-12.4227, -76.486)
  line L5009 (-12.4227, -76.486) -> (-12.5142, -76.6472)
  line L5010 (-20.2813, -75.437) -> (-20.2924, -75.1547)
  line L5011 (-13.0995, -75.169) -> (-12.9224, -75.2239)
  line L5012 (-19.8542, -76.468) -> (-20.0148, -76.2356)
  line L5013 (-13.6709, -76.9702) -> (-13.8327, -76.8797)
  line L5014 (-19.9475, -74.0933) -> (-19.7726, -73.8715)
  line L5015 (-18.2619, -73.2177) -> (-17.9805, -73.2421)
  line L5016 (-14.0744, -75.5629) -> (-13.9552, -75.4209)
  line L5017 (172.942, -74.7575) -> (172.962, -74.93)
  line L5018 (-18.8211, -73.2884) -> (-18.544, -73.2333)
  line L5019 (172.962, -74.93) -> (172.962, -75.93)
  line L5020 (-13.4945, -77.0275) -> (-13.6709, -76.9702)
  line L5021 (-12.9224, -75.2239) -> (-12.7593, -75.312)
  line L5022 (-12.7593, -75.312) -> (-12.6164, -75.4302)
  line L5023 (-12.3409, -76.1262) -> (-12.3641, -76.3101)
  line L5024 (-19.3383, -73.5122) -> (-19.0876, -73.382)
  line L5025 (-13.8327, -76.8797) -> (-13.9739, -76.7596)
  line L5026 (-19.2013, -76.9995) -> (-19.4434, -76.8538)
  line L5027 (172.956, -76.0227) -> (172.915, -76.1914)
  line L5028 (172.345, -74.1919) -> (172.511, -74.2422)
  line L5029 (-13.3104, -77.0494) -> (-13.4945, -77.0275)
  line L5030 (172.511, -74.2422) -> (172.661, -74.3295)
  line L5031 (-14.2404, -76.0864) -> (-14.2198, -75.9021)
  line L5032 (-20.0894, -74.3376) -> (-19.9475, -74.0933)
  line L5033 (-13.9552, -75.4209) -> (-13.8107, -75.3047)
  line L5034 (-12.947, -76.9853) -> (-13.1256, -77.0352)
  line L5035 (-13.8107, -75.3047) -> (-13.6464, -75.2188)
  line L5036 (-13.4685, -75.1665) -> (-13.2839, -75.1497)
  line L5037 (-14.2249, -76.2711) -> (-14.2404, -76.0864)
  line L5038 (-12.4122, -75.7376) -> (-12.3586, -75.9151)
  line L5039 (-12.7815, -76.9017) -> (-12.947, -76.9853)
  line L5040 (-20.1955, -74.5995) -> (-20.0894, -74.3376)
  line L5041 (-12.5142, -76.6472) -> (-12.6354, -76.7876)
  line L5042 (-13.9739, -76.7596) -> (-14.0891, -76.6143)
  line L5043 (172.962, -75.93) -> (172.956, -76.0227)
  line L5044 (-19.0876, -73.382) -> (-18.8211, -73.2884)
  line L5045 (-12.4992, -75.5739) -> (-12.4122, -75.7376)
  line L5046 (-19.4434, -76.8538) -> (-19.6624, -76.6754)
  line L5047 (172.883, -74.5942) -> (172.942, -74.7575)
  line L5048 (-19.6624, -76.6754) -> (-19.8542, -76.468)
  line L5049 (-20.2636, -74.8736) -> (-20.1955, -74.5995)
  line L5050 (-12.6354, -76.7876) -> (-12.7815, -76.9017)
  line L5051 (-14.2198, -75.9021) -> (-14.1637, -75.7254)
  line L5052 (-20.0148, -76.2356) -> (-20.1411, -75.9829)
  line L5053 (172.787, -74.4489) -> (172.883, -74.5942)
  line L5054 (-14.1637, -75.7254) -> (-14.0744, -75.5629)
  line L5055 (172.915, -76.1914) -> (172.836, -76.3461)
  line L5056 (-14.1738, -76.4493) -> (-14.2249, -76.2711)
  line L5057 (171.468, -74.8373) -> (171.509, -74.6686)
  line L5058 (169.884, -76.6495) -> (169.713, -76.6789)
  line L5059 (172.661, -74.3295) -> (172.787, -74.4489)
  line L5060 (172, -74.2105) -> (172.171, -74.1811)
  line L5061 (169.048, -74.5139) -> (169.161, -74.3815)
  line L5062 (168.942, -76.1025) -> (168.922, -75.93)
  line L5063 (171.541, -76.2658) -> (171.482, -76.1025)
  line L5064 (171.509, -74.6686) -> (171.588, -74.5139)
  line L5065 (169.631, -74.1811) -> (169.805, -74.1919)
  line L5066 (171.763, -76.5305) -> (171.637, -76.4111)
  line L5067 (169.539, -76.6681) -> (169.373, -76.6178)
  line L5068 (169.373, -76.6178) -> (169.223, -76.5305)
  line L5069 (167.756, -76.3461) -> (167.643, -76.4785)
  line L5070 (167.835, -76.1914) -> (167.756, -76.3461)
  line L5071 (172.171, -74.1811) -> (172.345, -74.1919)
  line L5072 (168.922, -75.93) -> (168.922, -74.93)
  line L5073 (167.344, -76.6495) -> (167.173, -76.6789)
  line L5074 (172.836, -76.3461) -> (172.723, -76.4785)
  line L5075 (-13.2839, -75.1497) -> (-13.0995, -75.169)
  line L5076 (172.723, -76.4785) -> (172.584, -76.5815)
  line L5077 (170.247, -74.4489) -> (170.343, -74.5942)
  line L5078 (167.581, -74.3295) -> (167.707, -74.4489)
  line L5079 (170.044, -76.5815) -> (169.884, -76.6495)
  line L5080 (168.928, -74.8373) -> (168.969, -74.6686)
  line L5081 (170.416, -76.0227) -> (170.375, -76.1914)
  line L5082 (170.296, -76.3461) -> (170.183, -76.4785)
  line L5083 (-14.0891, -76.6143) -> (-14.1738, -76.4493)
  line L5084 (167.882, -75.93) -> (167.876, -76.0227)
  line L5085 (168.922, -74.93) -> (168.928, -74.8373)
  line L5086 (-13.6464, -75.2188) -> (-13.4685, -75.1665)
  line L5087 (169.971, -74.2422) -> (170.121, -74.3295)
  line L5088 (171.462, -74.93) -> (171.468, -74.8373)
  line L5089 (167.803, -74.5942) -> (167.862, -74.7575)
  line L5090 (171.462, -75.93) -> (171.462, -74.93)
  line L5091 (168.969, -74.6686) -> (169.048, -74.5139)
  line L5092 (167.265, -74.1919) -> (167.431, -74.2422)
  line L5093 (167.882, -74.93) -> (167.882, -75.93)
  line L5094 (170.343, -74.5942) -> (170.402, -74.7575)
  line L5095 (170.402, -74.7575) -> (170.422, -74.93)
  line L5096 (172.424, -76.6495) -> (172.253, -76.6789)
  line L5097 (167.431, -74.2422) -> (167.581, -74.3295)
  line L5098 (169.223, -76.5305) -> (169.097, -76.4111)
  line L5099 (169.46, -74.2105) -> (169.631, -74.1811)
  line L5100 (167.862, -74.7575) -> (167.882, -74.93)
  line L5101 (167.876, -76.0227) -> (167.835, -76.1914)
  line L5102 (169.161, -74.3815) -> (169.3, -74.2785)
  line L5103 (167.643, -76.4785) -> (167.504, -76.5815)
  line L5104 (169.097, -76.4111) -> (169.001, -76.2658)
  line L5105 (172.079, -76.6681) -> (171.913, -76.6178)
  line L5106 (171.588, -74.5139) -> (171.701, -74.3815)
  line L5107 (-13.1256, -77.0352) -> (-13.3104, -77.0494)
  line L5108 (171.84, -74.2785) -> (172, -74.2105)
  line L5109 (170.121, -74.3295) -> (170.247, -74.4489)
  line L5110 (170.422, -75.93) -> (170.416, -76.0227)
  line L5111 (169.805, -74.1919) -> (169.971, -74.2422)
  line L5112 (172.584, -76.5815) -> (172.424, -76.6495)
  line L5113 (170.375, -76.1914) -> (170.296, -76.3461)
  line L5114 (171.637, -76.4111) -> (171.541, -76.2658)
  line L5115 (172.253, -76.6789) -> (172.079, -76.6681)
  line L5116 (171.701, -74.3815) -> (171.84, -74.2785)
  line L5117 (171.913, -76.6178) -> (171.763, -76.5305)
  line L5118 (170.422, -74.93) -> (170.422, -75.93)
  line L5119 (171.482, -76.1025) -> (171.462, -75.93)
  line L5120 (170.183, -76.4785) -> (170.044, -76.5815)
  line L5121 (166.382, -74.93) -> (166.388, -74.8373)
  line L5122 (169.001, -76.2658) -> (168.942, -76.1025)
  line L5123 (165.103, -76.4785) -> (164.964, -76.5815)
  line L5124 (166.833, -76.6178) -> (166.683, -76.5305)
  line L5125 (164.459, -76.6681) -> (164.293, -76.6178)
  line L5126 (169.713, -76.6789) -> (169.539, -76.6681)
  line L5127 (166.557, -76.4111) -> (166.461, -76.2658)
  line L5128 (165.336, -76.0227) -> (165.295, -76.1914)
  line L5129 (165.295, -76.1914) -> (165.216, -76.3461)
  line L5130 (169.3, -74.2785) -> (169.46, -74.2105)
  line L5131 (166.382, -75.93) -> (166.382, -74.93)
  line L5132 (167.173, -76.6789) -> (166.999, -76.6681)
  line L5133 (163.889, -74.6686) -> (163.968, -74.5139)
  line L5134 (164.293, -76.6178) -> (164.143, -76.5305)
  line L5135 (163.842, -75.93) -> (163.842, -74.93)
  line L5136 (167.504, -76.5815) -> (167.344, -76.6495)
  line L5137 (164.964, -76.5815) -> (164.804, -76.6495)
  line L5138 (166.621, -74.3815) -> (166.76, -74.2785)
  line L5139 (162.563, -76.4785) -> (162.424, -76.5815)
  line L5140 (163.862, -76.1025) -> (163.842, -75.93)
  line L5141 (162.264, -76.6495) -> (162.093, -76.6789)
  line L5142 (164.804, -76.6495) -> (164.633, -76.6789)
  line L5143 (162.424, -76.5815) -> (162.264, -76.6495)
  line L5144 (161.753, -76.6178) -> (161.603, -76.5305)
  line L5145 (162.627, -74.4489) -> (162.723, -74.5942)
  line L5146 (163.848, -74.8373) -> (163.889, -74.6686)
  line L5147 (163.968, -74.5139) -> (164.081, -74.3815)
  line L5148 (162.185, -74.1919) -> (162.351, -74.2422)
  line L5149 (165.342, -75.93) -> (165.336, -76.0227)
  line L5150 (165.041, -74.3295) -> (165.167, -74.4489)
  line L5151 (167.707, -74.4489) -> (167.803, -74.5942)
  line L5152 (164.891, -74.2422) -> (165.041, -74.3295)
  line L5153 (164.633, -76.6789) -> (164.459, -76.6681)
  line L5154 (165.216, -76.3461) -> (165.103, -76.4785)
  line L5155 (162.723, -74.5942) -> (162.782, -74.7575)
  line L5156 (161.603, -76.5305) -> (161.477, -76.4111)
  line L5157 (162.802, -74.93) -> (162.802, -75.93)
  line L5158 (164.38, -74.2105) -> (164.551, -74.1811)
  line L5159 (166.461, -76.2658) -> (166.402, -76.1025)
  line L5160 (166.76, -74.2785) -> (166.92, -74.2105)
  line L5161 (166.683, -76.5305) -> (166.557, -76.4111)
  line L5162 (162.351, -74.2422) -> (162.501, -74.3295)
  line L5163 (164.143, -76.5305) -> (164.017, -76.4111)
  line L5164 (164.22, -74.2785) -> (164.38, -74.2105)
  line L5165 (167.091, -74.1811) -> (167.265, -74.1919)
  line L5166 (166.429, -74.6686) -> (166.508, -74.5139)
  line L5167 (165.263, -74.5942) -> (165.322, -74.7575)
  line L5168 (164.725, -74.1919) -> (164.891, -74.2422)
  line L5169 (162.782, -74.7575) -> (162.802, -74.93)
  line L5170 (162.676, -76.3461) -> (162.563, -76.4785)
  line L5171 (163.842, -74.93) -> (163.848, -74.8373)
  line L5172 (162.093, -76.6789) -> (161.919, -76.6681)
  line L5173 (162.755, -76.1914) -> (162.676, -76.3461)
  line L5174 (161.919, -76.6681) -> (161.753, -76.6178)
  line L5175 (162.796, -76.0227) -> (162.755, -76.1914)
  line L5176 (162.501, -74.3295) -> (162.627, -74.4489)
  line L5177 (165.342, -74.93) -> (165.342, -75.93)
  line L5178 (165.167, -74.4489) -> (165.263, -74.5942)
  line L5179 (165.322, -74.7575) -> (165.342, -74.93)
  line L5180 (166.402, -76.1025) -> (166.382, -75.93)
  line L5181 (166.92, -74.2105) -> (167.091, -74.1811)
  line L5182 (166.508, -74.5139) -> (166.621, -74.3815)
  line L5183 (166.388, -74.8373) -> (166.429, -74.6686)
  line L5184 (166.999, -76.6681) -> (166.833, -76.6178)
  line L5185 (161.302, -75.93) -> (161.302, -74.93)
  line L5186 (174.203, -75.4415) -> (174.101, -75.3016)
  line L5187 (159.848, -75.6006) -> (159.685, -75.6599)
  line L5188 (174.752, -75.68) -> (174.659, -75.6742)
  line L5189 (174.101, -75.3016) -> (174.033, -75.1418)
  line L5190 (159.512, -75.68) -> (158.512, -75.68)
  line L5191 (176.233, -75.5054) -> (176.088, -75.6006)
  line L5192 (176.353, -75.3793) -> (176.233, -75.5054)
  line L5193 (174.336, -75.554) -> (174.203, -75.4415)
  line L5194 (159.605, -74.1858) -> (159.773, -74.227)
  line L5195 (176.013, -74.227) -> (176.168, -74.306)
  line L5196 (162.802, -75.93) -> (162.796, -76.0227)
  line L5197 (157.861, -75.3016) -> (157.793, -75.1418)
  line L5198 (160.231, -74.7182) -> (160.261, -74.8894)
  line L5199 (176.403, -74.5584) -> (176.471, -74.7182)
  line L5200 (176.44, -75.2291) -> (176.353, -75.3793)
  line L5201 (161.308, -74.8373) -> (161.349, -74.6686)
  line L5202 (161.349, -74.6686) -> (161.428, -74.5139)
  line L5203 (158.512, -75.68) -> (158.419, -75.6742)
  line L5204 (161.322, -76.1025) -> (161.302, -75.93)
  line L5205 (164.017, -76.4111) -> (163.921, -76.2658)
  line L5206 (176.168, -74.306) -> (176.301, -74.4185)
  line L5207 (164.081, -74.3815) -> (164.22, -74.2785)
  line L5208 (163.921, -76.2658) -> (163.862, -76.1025)
  line L5209 (160.113, -75.3793) -> (159.993, -75.5054)
  line L5210 (164.551, -74.1811) -> (164.725, -74.1919)
  line L5211 (174.752, -74.18) -> (175.752, -74.18)
  line L5212 (175.752, -74.18) -> (175.845, -74.1858)
  line L5213 (159.993, -75.5054) -> (159.848, -75.6006)
  line L5214 (161.477, -76.4111) -> (161.381, -76.2658)
  line L5215 (159.685, -75.6599) -> (159.512, -75.68)
  line L5216 (160.261, -74.8894) -> (160.25, -75.0628)
  line L5217 (160.163, -74.5584) -> (160.231, -74.7182)
  line L5218 (157.963, -75.4415) -> (157.861, -75.3016)
  line L5219 (157.763, -74.9706) -> (157.774, -74.7972)
  line L5220 (176.088, -75.6006) -> (175.925, -75.6599)
  line L5221 (162.011, -74.1811) -> (162.185, -74.1919)
  line L5222 (160.25, -75.0628) -> (160.2, -75.2291)
  line L5223 (159.928, -74.306) -> (160.061, -74.4185)
  line L5224 (174.659, -75.6742) -> (174.491, -75.633)
  line L5225 (174.579, -74.2001) -> (174.752, -74.18)
  line L5226 (174.064, -74.6309) -> (174.151, -74.4807)
  line L5227 (161.84, -74.2105) -> (162.011, -74.1811)
  line L5228 (160.2, -75.2291) -> (160.113, -75.3793)
  line L5229 (174.151, -74.4807) -> (174.271, -74.3546)
  line L5230 (174.491, -75.633) -> (174.336, -75.554)
  line L5231 (176.501, -74.8894) -> (176.49, -75.0628)
  line L5232 (176.49, -75.0628) -> (176.44, -75.2291)
  line L5233 (161.381, -76.2658) -> (161.322, -76.1025)
  line L5234 (161.541, -74.3815) -> (161.68, -74.2785)
  line L5235 (160.061, -74.4185) -> (160.163, -74.5584)
  line L5236 (157.793, -75.1418) -> (157.763, -74.9706)